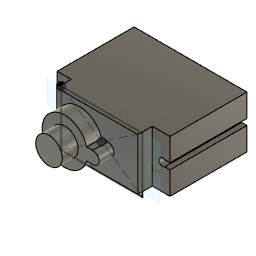
SERVO MOTOR SG90 v1 (Autodesk Fusion 360 design; units mm, degrees)
Autodesk Fusion 360 part; units mm, degrees
sketch "Sketch1" plane through (0, 0, 0) normal (0, 1, 0) x (1, 0, 0)
  line L0 (16, -7.35) -> (-16, -7.35)
  line L1 (-16, -7.35) -> (-16, 7.35)
  line L2 (-16, 7.35) -> (16, 7.35)
  line L3 (16, 7.35) -> (16, -7.35)
  line L4 (16, -7.35) -> (-16, 7.35) construction
  line L5 (-16, -7.35) -> (16, 7.35) construction
  circle A0 centre (13.9, 0) radius 1.05
  line L6 (0, 0) -> (16, 0)
  line L7 (14.4751, -0.8785) -> (16, -0.8785)
  line L8 (0, 0) -> (0, -1.4993)
  line L9 (0, -1.4993) -> (0, -7.35)
  line L10 (-14.4751, -0.8785) -> (-16, -0.8785)
  circle A1 centre (-13.9, 0) radius 1.05
  line L11 (0, -1.4993) -> (0, -7.35)
  line L12 (0, 0) -> (0, -1.4993)
  line L13 (-16, 1) -> (-14.2202, 1)
  line L14 (14.5262, 0.8429) -> (16, 0.8429)
  dimension "d1" = 32
  dimension "d2" = 14.7
  dimension "d3" = 2.1
  dimension "d4" = 2.1
  dimension "d6" = 1.5249
  dimension "d7" = 1.5249
  constraint horizontal L0
  constraint perpendicular L0 L1
  constraint parallel L0 L2
  constraint parallel L1 L3
  constraint coincident L4 L6.start
  constraint coincident L5 L6.start
  constraint coincident L6.start L8.start
  constraint midpoint L3 L6.end
  constraint coincident A0 L7.start
  constraint coincident L3 L7.end
  constraint perpendicular L3 L7
  constraint perpendicular L6 L8
  constraint midpoint L0 L9.end
  constraint perpendicular L0 L9
  constraint symmetric A0 L9 A1
  constraint symmetric L7.start L9 L10.start
  constraint symmetric L7.end L9 L10.end
  constraint symmetric L6.start L9 L8.start
  constraint symmetric L8.end L9 L11.start
  constraint symmetric L11.end L9 L9.end
  constraint coincident L1 L13.start
  constraint coincident A1 L13.end
  constraint perpendicular L1 L13
  constraint coincident A0 L14.start
  constraint coincident L3 L14.end
  constraint perpendicular L3 L14
  measures "d1" distance of L0.start L0.end
  measures "d2" distance of L0.end L1.end
  measures "d3" diameter of A0
  measures "d4" distance of L3 A0.centre
  measures "d6" distance of L7.start L7.end
  measures "d7" distance of L7.start L7.end
extrude "Extrude1" add sketch "Sketch1" along normal blind 2.3 contours L0 L3 A0 L6 L7 L8 L9 L11 L12 | L0 L1 L2 L3 A0 L6 L8 L9 L10 A1 L11 L12 L13 L14 in component "Component"
sketch "Sketch2" plane through (0, 0.4968, 0) normal (0, -1, 0) x (1, 0, 0)
  arc A0 (15.0024, 1.3496) -> (15.0535, -0.3718) centre (14.4273, 0.4711) ccw
  line L0 (15.0024, 1.3496) -> (16.5273, 1.3496)
  line L1 (16.5273, 1.3496) -> (16.5273, 7.8211)
  line L2 (16.5273, 7.8211) -> (-15.4727, 7.8211)
  line L3 (-15.4727, 7.8211) -> (-15.4727, 1.3496)
  line L4 (-15.4727, 1.3496) -> (-13.9478, 1.3496)
  arc A1 (-13.6929, -0.5289) -> (-13.9478, 1.3496) centre (-13.3727, 0.4711) ccw
  line L5 (-13.6929, -0.5289) -> (-15.4727, -0.5289)
  line L6 (-15.4727, -0.5289) -> (-15.4727, -6.8789)
  line L7 (-15.4727, -6.8789) -> (16.5273, -6.8789)
  line L8 (16.5273, -6.8789) -> (16.5273, -0.3718)
  line L9 (16.5273, -0.3718) -> (15.0535, -0.3718)
  line L10 (-11.5, 7.8211) -> (11.5, 7.8211)
  line L11 (11.5, 7.8211) -> (11.5, -7.8211)
  line L12 (11.5, -7.8211) -> (-11.5, -7.8211)
  line L13 (-11.5, -7.8211) -> (-11.5, 7.8211)
  line L14 (-11.5, 7.8211) -> (11.5, -7.8211) construction
  line L15 (11.5, 7.8211) -> (-11.5, -7.8211) construction
  dimension "d14" = 15.6422
  dimension "d15" = 23
  constraint horizontal L10
  constraint perpendicular L10 L11
  constraint parallel L10 L12
  constraint parallel L11 L13
  constraint coincident L14 origin
  constraint coincident L15 origin
  constraint coincident L2 L10.start
  measures "d14" distance of L10.start L12.end
  measures "d15" distance of L11.end L12.end
sketch "Sketch3" plane through (0, 0.4968, 0) normal (0, -1, 0) x (1, 0, 0)
extrude "Extrude2" add sketch "Sketch2" along normal blind 4.1 contours L2 L7 L10 L11 L13 sketch seen with x (1, 0, 0) y (0, 1, 0) z (0, 0, 1) at (-0.5273, -0.4968, -0.4711) in component "Component"
sketch "Sketch4" plane through (0, -3.6032, 0) normal (0, -1, 0) x (1, 0, 0)
  line L0 (-11.5, 7.8211) -> (-11.5, -6.8789)
  line L1 (-11.5, -6.8789) -> (11.5, -6.8789)
  line L2 (11.5, -6.8789) -> (11.5, 7.8211)
  line L3 (11.5, 7.8211) -> (-11.5, 7.8211)
  line L4 (0, 0) -> (-23, 0)
  line L5 (-23, 0) -> (0, 0)
  line L6 (2.8707, 1.7263) -> (1.1969, 1.7263)
  line L7 (2.8707, -1.7263) -> (1.1969, -1.7263)
  arc A0 (2.8707, -1.7263) -> (2.8707, 1.7263) centre (3, 0) ccw
  arc A1 (1.1969, 1.7263) -> (1.1969, -1.7263) centre (-5, 0) ccw
  dimension "d18" = 3
  constraint coincident L4.start L5.end
  constraint perpendicular L0 L4
  constraint coincident L4 A1.centre
  constraint symmetric L4 L6.start L7.start
  constraint horizontal L6
  measures "d18" distance of L4.start A0.centre
extrude "Extrude3" add sketch "Sketch4" along normal blind 4.2 contours L6 L7 A0 A1 sketch seen with x (1, 0, 0) y (0, 1, 0) z (0, 0, 1) at (-0.5273, -0.4968, -0.4711) in component "Component"
sketch "Sketch5" plane through (0, 2.7968, 0) normal (0, 1, 0) x (-1, 0, 0)
  arc A0 (-15.0535, -0.3718) -> (-15.0024, 1.3496) centre (-14.4273, 0.4711) ccw
  line L0 (-15.0535, -0.3718) -> (-16.5273, -0.3718)
  line L1 (-16.5273, -0.3718) -> (-16.5273, -6.8789)
  line L2 (-16.5273, -6.8789) -> (15.4727, -6.8789)
  line L3 (15.4727, -6.8789) -> (15.4727, -0.5289)
  line L4 (15.4727, -0.5289) -> (13.6929, -0.5289)
  arc A1 (13.9478, 1.3496) -> (13.6929, -0.5289) centre (13.3727, 0.4711) ccw
  line L5 (13.9478, 1.3496) -> (15.4727, 1.3496)
  line L6 (15.4727, 1.3496) -> (15.4727, 7.8211)
  line L7 (15.4727, 7.8211) -> (-16.5273, 7.8211)
  line L8 (-16.5273, 7.8211) -> (-16.5273, 1.3496)
  line L9 (-16.5273, 1.3496) -> (-15.0024, 1.3496)
sketch "Sketch6" plane through (0, 2.7968, 0) normal (0, 1, 0) x (-1, 0, 0)
sketch "Sketch7" plane through (0, 0.4968, 0) normal (0, -1, 0) x (1, 0, 0)
extrude "Extrude4" add sketch "Sketch5" along normal blind 19.5 sketch seen with x (1, 0, 0) y (0, 1, 0) z (0, 0, 1) at (-0.5273, -0.4968, -0.4711) in component "Component"
sketch "Sketch8" plane through (0, 0.4968, 0) normal (0, -1, 0) x (1, 0, 0)
sketch "Sketch9" plane through (0, -7.8032, 0) normal (0, -1, 0) x (1, 0, 0)
  arc A0 (2.8707, -1.7263) -> (2.8707, 1.7263) centre (3, 0) ccw
  line L0 (2.8707, 1.7263) -> (1.1969, 1.7263)
  arc A1 (1.1969, 1.7263) -> (1.1969, -1.7263) centre (-5, 0) ccw
  line L1 (1.1969, -1.7263) -> (2.8707, -1.7263)
  circle A2 centre (-5, 0) radius 3.7758
  constraint concentric A1 A2
extrude "Extrude5" add sketch "Sketch9" along normal blind 4.5 contours A2 sketch seen with x (1, 0, 0) y (0, 1, 0) z (0, 0, 1) at (-0.5273, -0.4968, -0.4711) in component "Component"
component "Component" placed x (1, 0, 0) y (0, 1, 0) z (0, 0, 1) at (0.5273, 0.4968, 0.4711)
